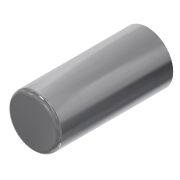
# Autodesk Inventor part: PP-15
Saved by Autodesk Inventor 2022 (Build 260148000, 148)
## iProperties
Created: 2008-09-23
Part Number: PP-15
Document SubType Name: Modeling
Designer: Mark Flayler
Mass: 1.1664 g
Surface Area: 5.5153 cm^2
Volume: 0.148586 cm^3
Density: 7.85 g/cm^3
Material: Steel
Description: ERASER CAP
Appearance: Aluminum - Polished
Author: Mark Flayler
Autodesk Inventor part; units mm, degrees
ref_plane "YZ Plane" through (0, 0, 0) normal (1, 0, 0) x (0, 1, 0)
ref_plane "XZ Plane" through (0, 0, 0) normal (0, 1, 0) x (-1, 0, 0)
ref_plane "XY Plane" through (0, 0, 0) normal (0, 0, 1) x (1, 0, 0)
sketch "Sketch1" plane through (0, 0, 0) normal (0, 0, 1) x (1, 0, 0)
  line L0 (0, 0) -> (0, 14)
  line L1 (0, 0) -> (0, 1)
  line L2 (0, 1) -> (2.65, 1)
  line L3 (2.65, 1) -> (2.65, 14)
  line L4 (2.65, 14) -> (3.15, 14)
  line L5 (3.15, 14) -> (3.15, 0)
  line L6 (3.15, 0) -> (0, 0)
  dimension "d0" = 5.3
  dimension "d1" = 6.3
  dimension "d2" = 13
  dimension "d3" = 14
  constraints: 14 end point, 3 parallel, 2 perpendicular, 1 horizontal alignment, 1 point on line, 1 vertical
  measures "d0" diameter of L3 L0
  measures "d1" diameter of L5 L0
  measures "d2" distance between parallel lines of L2 L4
  measures "d3" distance between parallel lines of L6 L4
revolve "Revolution1" add sketch "Sketch1" angle 360 about axis through (0, 0, 0) along (0, 1, 0)
fillet "Fillet1" radius 0.5 1 edges at (-3.15, 0, 0)
body "Solid1"
